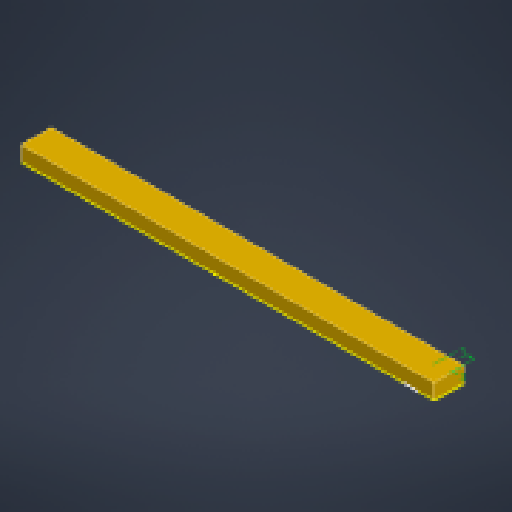
# Autodesk Inventor part: Slider
Saved by Autodesk Inventor 2023 (Build 270158000, 158)
## iProperties
Created: 2023-05-08
Part Number: Slider
Material: Generic
Document SubType Name: Modeling
Designer: szykr
Density: 1 g/cm^3
Appearance: Gold
Author: szykr
Autodesk Inventor part; units mm, degrees
ref_plane "YZ Plane" through (0, 0, 0) normal (1, 0, 0) x (0, 1, 0)
ref_plane "XZ Plane" through (0, 0, 0) normal (0, 1, 0) x (-1, 0, 0)
ref_plane "XY Plane" through (0, 0, 0) normal (0, 0, 1) x (1, 0, 0)
sketch "Sketch1" plane through (0, 0, 0) normal (0, 1, 0) x (-1, 0, 0)
  line L0 (-4.6, -6) -> (-4.6, 0) projected
  line L1 (0, -6) -> (-4.6, -6) projected
  line L2 (0, 0) -> (0, -6) projected
  line L3 (0, 0) -> (-4.6, 0) projected
  line L4 (37.7, -0.1) -> (-42.3, -0.1)
  line L5 (-42.3, -0.1) -> (-42.3, -5.9)
  line L6 (-42.3, -5.9) -> (37.7, -5.9)
  line L7 (37.7, -5.9) -> (37.7, -0.1)
  line L8 (-2.3, -6) -> (-2.3, 0) construction
  dimension "d0" = 0.1
  dimension "d1" = 0.1
  dimension "d2" = 80
  constraints: 10 end point, 2 midpoint, 2 parallel, 1 horizontal, 1 perpendicular, 1 other
  measures "d0" distance between parallel lines of L3 L4
  measures "d1" distance between parallel lines of L1 L6
  measures "d2" distance between parallel lines of L5 L7
extrude "Extrusion1" add sketch "Sketch1" along normal blind 2.9 contours L6 L5 L4 L0 | L0 L4 L2 L6 | L2 L4 L7 L6
sketch "Sketch3" plane through (0, 0, 0) normal (0, -1, 0) x (1, 0, 0)
  line L0 (42.3, -5.9) -> (-37.7, -5.9) projected
  line L1 (-37.7, -0.1) -> (42.3, -0.1) projected
  line L2 (39.3, -5.9) -> (36.3, -5.9)
  line L3 (36.3, -5.9) -> (36.3, -0.1)
  line L4 (36.3, -0.1) -> (39.3, -0.1)
  line L5 (39.3, -0.1) -> (39.3, -5.9)
  line L6 (39.3, -4.5) -> (36.3, -4.5)
  line L7 (36.3, -4.5) -> (36.3, -1.5)
  line L8 (36.3, -1.5) -> (39.3, -1.5)
  line L9 (39.3, -1.5) -> (39.3, -4.5)
  line L10 (39.3, -3) -> (36.3, -3) construction
  line L11 (42.3, -0.1) -> (42.3, -5.9) projected
  point P0 (0, 0)
  dimension "d5" = 3
  dimension "d6" = 3
  constraints: 18 end point, 4 parallel, 3 perpendicular, 2 collinear, 2 horizontal, 2 midpoint, 2 point on line, 1 other
  measures "d5" distance between parallel lines of L5 L3
  measures "d6" distance between parallel lines of L11 L5
extrude "Extrusion2" cut sketch "Sketch3" against normal through all contours L6 L3 L8 L5
extrude "Extrusion3" cut sketch "Sketch3" against normal blind 1.5 contours L0 L3 L6 L5 | L5 L8 L3 L1
pattern_linear "Rectangular Pattern1" count 5 spacing 6 along (-1, 0, 0) of "Extrusion3", "Extrusion2"
ref_plane "Work Plane1" through (2.3, 0, -0.1) normal (1, 0, 0) x (0, 0, -1)
mirror "Mirror1" about plane through (2.3, 0, -0.1) normal (1, 0, 0) of "Extrusion3", "Extrusion2", "Rectangular Pattern1"
equation "\"d0\" = slack"
equation "\"d1\" = slack"
equation "\"slack\" = 0.1"
body "Solid1"
